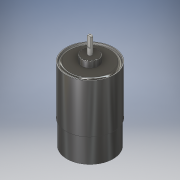
# Autodesk Inventor part: motor
Saved by Autodesk Inventor 2016 (Build 200138000, 138)
## iProperties
Created: 2018-01-02
Part Number: motor
Material: Generic
Document SubType Name: Modeling
Designer: student
Density: 1 g/cm^3
Appearance: Default
Author: student
Autodesk Inventor part; units mm, degrees
ref_plane "YZ Plane" through (0, 0, 0) normal (1, 0, 0) x (0, 1, 0)
ref_plane "XZ Plane" through (0, 0, 0) normal (0, 1, 0) x (-1, 0, 0)
ref_plane "XY Plane" through (0, 0, 0) normal (0, 0, 1) x (1, 0, 0)
sketch "Sketch1" plane through (0, 0, 0) normal (0, 1, 0) x (-1, 0, 0)
  circle A0 centre (0, 0) radius 17.907
  dimension "d0" = 35.814
  constraints: 1 centre point, 1 coincident
  measures "d0" diameter of A0
extrude "Extrusion1" add sketch "Sketch1" along normal blind 56.642
sketch "Sketch2" plane through (0, 56.642, 0) normal (0, 1, 0) x (1, 0, 0)
  circle A0 centre (0, 0) radius 6.5405
  dimension "d3" = 13.081
  constraints: 1 centre point, 1 coincident
  measures "d3" diameter of A0
extrude "Extrusion2" add sketch "Sketch2" along normal blind 4.826
sketch "Sketch3" plane through (0, 61.468, 0) normal (0, 1, 0) x (1, 0, 0)
  circle A0 centre (0, 0) radius 1.6256
  dimension "d6" = 3.2512
  constraints: 1 centre point, 1 coincident
  measures "d6" diameter of A0
extrude "Extrusion3" add sketch "Sketch3" along normal blind 5.08
sketch "Sketch4" plane through (0, 66.548, 0) normal (0, 1, 0) x (1, 0, 0)
  line L0 (-1.2863, -0.994) -> (1.2863, -0.994)
  arc A0 (1.2863, -0.994) -> (-1.2863, -0.994) centre (0, 0) ccw
  constraints: 2 end point, 2 point on circle, 1 centre point, 1 horizontal
extrude "Extrusion4" add sketch "Sketch4" along normal blind 8.128
fillet "Fillet1" radius 1.27 1 edges at (0, 74.676, -1.6256)
fillet "Fillet2" radius 2.54 1 edges at (17.907, 56.642, 0)
fillet "Fillet3" radius 0.508 1 edges at (-6.5405, 61.468, 0)
sketch "Sketch5" plane through (0, 56.642, 0) normal (0, 1, 0) x (1, 0, 0)
  circle A0 centre (0, 0) radius 0.3556 projected
  circle A1 centre (0, 0) radius 6.0325 projected
  circle A2 centre (0, 0) radius 18.542
  circle A3 centre (0, 0) radius 17.907
  dimension "d17" = 35.814
  dimension "d18" = 0.635
  constraints: 2 centre point, 2 coincident
  measures "d17" diameter of A3
  measures "d18" radial gap between concentric circles of A3 A2
extrude "Extrusion5" add sketch "Sketch5" against normal blind 37.7952 contours A2
body "Solid1"
